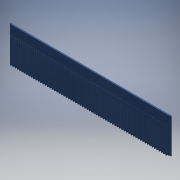
# Autodesk Inventor part: 99-445-27
Saved by Autodesk Inventor 2018 (Build 220105000, 105)
## iProperties
Created: 2004-11-23
Part Number: 99-445-27
Document SubType Name: Modeling
Designer: Autodesk, Inc.
Manufacturer: Standard
Standards Organization: Custom
Description: ESD, SLOTS, LONG
Mass: 91.61 g
Surface Area: 699.021 cm^2
Volume: 91.61 cm^3
Density: 1 g/cm^3
Material: Generic
Appearance: Flaked Satin - Blue
CAGE: 1LJX3
Dept. ID: Product Design
Description #2: ---
Finish #1: ---
Finish #2: ---
Material ID: ---
Project Number: ---
Author: Autodesk, Inc.
Autodesk Inventor part; units mm, degrees
ref_plane "YZ Plane" through (0, 0, 0) normal (1, 0, 0) x (0, 1, 0)
ref_plane "XZ Plane" through (0, 0, 0) normal (0, 1, 0) x (-1, 0, 0)
ref_plane "XY Plane" through (0, 0, 0) normal (0, 0, 1) x (1, 0, 0)
sketch "Sketch1" plane through (0, 0, 0) normal (0, 0, 1) x (1, 0, 0)
  line L0 (-170, 37.5) -> (170, 37.5)
  line L1 (170, 37.5) -> (170, -37.5)
  line L2 (170, -37.5) -> (-170, -37.5)
  line L3 (-170, -37.5) -> (-170, 37.5)
  point P0 (0, 0)
  point P1 (-170, 0)
  point P2 (0, 37.5)
  dimension "d0" = 75
  dimension "d1" = 340
  constraints: 8 end point, 2 midpoint, 2 parallel, 1 horizontal, 1 horizontal alignment, 1 perpendicular, 1 vertical alignment
  measures "d0" distance of L2.end L0.start
  measures "d1" distance of L0.start L0.end
extrude "Extrusion1" add sketch "Sketch1" along normal blind 3
sketch "Sketch2" plane through (0, 0, 3) normal (0, 0, 1) x (1, 0, 0)
  line L0 (170, -37.5) -> (-170, -37.5) projected
  line L1 (-170, -37.5) -> (-170, 10)
  line L2 (-170, 10) -> (-169.375, 17.5)
  line L3 (-169.375, 17.5) -> (-168.625, 17.5)
  line L4 (-168.625, 17.5) -> (-168, 10)
  line L5 (-168, 10) -> (-168, -37.5)
  line L6 (-169, 17.5) -> (-169, -37.5) construction
  line L7 (-170, -37.5) -> (-170, 37.5) projected
  line L8 (-170, 37.5) -> (170, 37.5) projected
  dimension "d4" = 2
  dimension "d5" = 0.75
  dimension "d15" = 7.5
  dimension "d16" = 20
  constraints: 12 end point, 4 perpendicular, 3 point on line, 1 collinear, 1 midpoint, 2 other
  measures "d4" distance between parallel lines of L5 L1
  measures "d5" distance of L2.end L3.end
  measures "d15" distance from line of L1.end L3
  measures "d16" distance between parallel lines of L8 L3
extrude "Extrusion2" add sketch "Sketch2" along normal blind 2
pattern_linear "Rectangular Pattern1" count 68 spacing 5 along (1, 0, 0) of "Extrusion2"
sketch "Sketch3" plane through (170, -37.5, 0) normal (1, 0, 0) x (0, 0, -1)
  line L0 (0, 0) -> (-5, 0) projected
  line L1 (0, 75) -> (0, 0) projected
  line L2 (0, 75) -> (-3, 75) projected
  line L3 (-1.5, 75) -> (-1.5, 0)
  constraints: 2 end point, 1 midpoint, 1 parallel, 1 point on line
extrude "Extrusion3" add sketch "Sketch3" along normal blind 3.5
mirror "Mirror1" about plane through (0, 0, 0) normal (1, 0, 0) of "Extrusion3"
body "Solid1"
